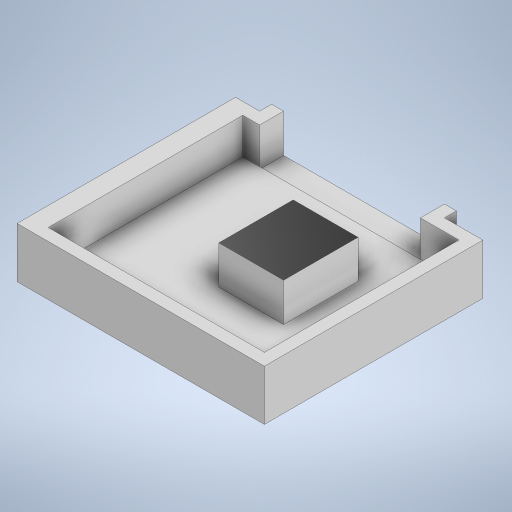
# Autodesk Inventor part: imu
Saved by Autodesk Inventor 2023 (Build 270158000, 158)
## iProperties
Created: 2024-02-07
Part Number: imu
Material: 일반
Document SubType Name: Modeling
Designer: ps737
Density: 1 g/cm^3
Appearance: 기본값
Author: ps737
Autodesk Inventor part; units mm, degrees
ref_plane "YZ Plane" through (0, 0, 0) normal (1, 0, 0) x (0, 1, 0)
ref_plane "XZ Plane" through (0, 0, 0) normal (0, 1, 0) x (-1, 0, 0)
ref_plane "XY Plane" through (0, 0, 0) normal (0, 0, 1) x (1, 0, 0)
sketch "스케치1" plane through (0, 0, 0) normal (0, 1, 0) x (-1, 0, 0)
  line L0 (103, 0) -> (93, 0)
  line L1 (0, 0) -> (0, -91)
  line L2 (0, -91) -> (103, -91)
  line L3 (103, -91) -> (103, 0)
  line L4 (93, -91) -> (93, -96)
  line L5 (93, -96) -> (16, -96)
  line L6 (16, -96) -> (16, -91)
  line L7 (93, 0) -> (0, 0)
  line L8 (103, -5) -> (0, -5)
  line L9 (5, 0) -> (5, -91)
  line L10 (0, -86) -> (103, -86)
  line L11 (95, 0) -> (95, -91)
  point P0 (93, -93.5)
  point P1 (16, -93.5)
  point P2 (51.5, -86)
  point P3 (95, -5)
  point P4 (95, -86)
  point P5 (5, -86)
  point P6 (5, -5)
  dimension "d0" = 103
  dimension "d1" = 91
  dimension "d2" = 5
  dimension "d3" = 10
  dimension "d4" = 16
  dimension "d5" = 8
  dimension "d6" = 5
  dimension "d7" = 5
  dimension "d8" = 5
  constraints: 24 end point, 11 point on line, 7 perpendicular, 4 parallel, 3 midpoint, 2 horizontal, 1 coincident, 1 vertical
  measures "d0" distance between parallel lines of L1 L3
  measures "d1" distance between parallel lines of L2 L0
  measures "d2" distance of L4.start L4.end
  measures "d3" distance from line of point (93, -93.5) L3
  measures "d4" distance from line of L1 point (16, -93.5)
  measures "d5" distance between parallel lines of L11 L3
  measures "d6" distance between parallel lines of L8 L7
  measures "d7" distance between parallel lines of L1 L9
  measures "d8" distance from line of L2 point (51.5, -86)
extrude "돌출1" add sketch "스케치1" along normal blind 21 contours L3 L8 L11 L0 | L11 L8 L9 L7 L0 | L3 L10 L11 L8 | L3 L2 L11 L10 | L9 L8 L1 L7 | L9 L10 L1 L8 | L11 L2 L9 L10 | L9 L2 L1 L10 | L4 L5 L6 L2
extrude "돌출2" add sketch "스케치1" along normal blind 6 contours L11 L10 L9 L8
sketch "스케치2" plane through (0, 21, 0) normal (0, 1, 0) x (1, 0, 0)
  line L0 (-16, 96) -> (-93, 96) projected
  line L1 (-21, 96) -> (-21, 86)
  line L2 (-95, 86) -> (-5, 86) projected
  line L3 (-88, 96) -> (-88, 76.7304)
  line L4 (-93, 96) -> (-93, 91) projected
  line L5 (-16, 91) -> (-16, 96) projected
  point P0 (0, 0)
  point P1 (-93, 93.5)
  point P2 (-88, 86)
  dimension "d13" = 5
  dimension "d14" = 5
  constraints: 4 end point, 3 point on line, 2 vertical, 1 midpoint
  measures "d13" distance from line of point (-93, 93.5) L3
  measures "d14" distance between parallel lines of L5 L1
extrude "돌출3" cut sketch "스케치2" against normal blind 16
sketch "스케치3" plane through (0, 6, 0) normal (0, 1, 0) x (1, 0, 0)
  line L0 (-95, 5) -> (-95, 86) projected
  line L1 (-95, 34) -> (-4.4574, 34)
  line L2 (-5, 86) -> (-5, 5) projected
  line L3 (-5, 65) -> (-95, 65)
  line L4 (-5, 5) -> (-95, 5) projected
  line L5 (-5, 5) -> (-95, 5) projected
  line L6 (-53, 5) -> (-53, 65)
  line L7 (-26, 5) -> (-26, 65)
  line L8 (-95, 5) -> (-95, 86) projected
  point P0 (0, 0)
  point P1 (-95, 45.5)
  point P2 (-26, 34)
  point P3 (-53, 34)
  dimension "d17" = 29
  dimension "d18" = 60
  dimension "d19" = 42
  dimension "d20" = 69
  constraints: 8 end point, 7 point on line, 3 perpendicular, 1 horizontal, 1 midpoint
  measures "d17" distance between parallel lines of L1 L4
  measures "d18" distance between parallel lines of L3 L4
  measures "d19" distance from line of point (-95, 45.5) L6
  measures "d20" distance between parallel lines of L0 L7
extrude "돌출4" add sketch "스케치3" along normal blind 16 contours L6 L3 L7 L1
